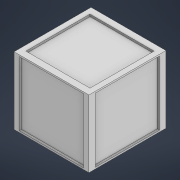
# Autodesk Inventor part: End-Effector
Saved by Autodesk Inventor 2022 (Build 260153000, 153)
## iProperties
Created: 2023-04-20
Part Number: End-Effector
Material: Generic
Document SubType Name: Modeling
Designer: Karl
Density: 1 g/cm^3
Appearance: Default
Author: Karl
Autodesk Inventor part; units mm, degrees
ref_plane "YZ Plane" through (0, 0, 0) normal (1, 0, 0) x (0, 1, 0)
ref_plane "XZ Plane" through (0, 0, 0) normal (0, 1, 0) x (-1, 0, 0)
ref_plane "XY Plane" through (0, 0, 0) normal (0, 0, 1) x (1, 0, 0)
sketch "Sketch3" plane through (0, 0, 0) normal (0, 0, 1) x (1, 0, 0)
  line L0 (0, 0) -> (-50, 0)
  line L1 (-50, 0) -> (-50, 43)
  line L2 (-50, 43) -> (0, 43)
  line L3 (0, 43) -> (0, 0)
  line L4 (10, -10) -> (-60, -10)
  line L5 (-60, -10) -> (-60, 53)
  line L6 (-60, 53) -> (10, 53)
  line L7 (10, 53) -> (10, -10)
  dimension "d26" = 43
  dimension "d27" = 50
  dimension "d28" = 70
  dimension "d29" = 63
  constraints: 16 end point, 4 parallel, 2 horizontal, 2 perpendicular
  measures "d26" distance of L2.end L0.start
  measures "d27" distance of L0.start L0.end
  measures "d28" distance of L5.end L6.end
  measures "d29" distance of L4.end L5.end
extrude "Extrusion3" add sketch "Sketch3" along normal blind 60
sketch "Sketch4" plane through (0, 0, 60) normal (0, 0, 1) x (1, 0, 0)
  line L0 (10, -10) -> (-60, -10)
  line L1 (-60, -10) -> (-60, 53)
  line L2 (-60, 53) -> (10, 53)
  line L3 (10, 53) -> (10, -10)
  point P0 (0, 0)
  constraints: 8 end point, 2 parallel, 1 horizontal, 1 perpendicular
extrude "Extrusion4" add sketch "Sketch4" along normal blind 12
sketch "Sketch5" plane through (-60, 53, 0) normal (0, 1, 0) x (1, 0, 0)
  line L0 (0, 0) -> (70, 0) projected
  line L1 (70, 0) -> (70, -72) projected
  line L2 (0, 0) -> (70, 0)
  line L3 (70, 0) -> (70, -72)
  line L4 (70, -72) -> (0, -72)
  line L5 (0, -72) -> (0, 0)
  line L6 (65, -6) -> (5, -6)
  line L7 (5, -6) -> (5, -66)
  line L8 (5, -66) -> (65, -66)
  line L9 (65, -66) -> (65, -6)
  line L10 (60, -11) -> (10, -11)
  line L11 (10, -11) -> (10, -61)
  line L12 (10, -61) -> (60, -61)
  line L13 (60, -61) -> (60, -11)
  point P0 (60, 0)
  dimension "d34" = 60
  dimension "d35" = 60
  dimension "d36" = 50
  dimension "d37" = 50
  constraints: 24 end point, 6 parallel, 3 horizontal, 3 perpendicular
  measures "d34" distance of L8.end L7.end
  measures "d35" distance of L7.end L6.end
  measures "d36" distance of L12.end L11.end
  measures "d37" distance of L11.end L10.end
extrude "Extrusion5" cut sketch "Sketch5" against normal blind 2 contours L9 L8 L7 L6 | L13 L12 L11 L10
sketch "Sketch6" plane through (10, -10, 0) normal (1, 0, 0) x (0, 0, -1)
  line L0 (-6, 1.5) -> (-66, 1.5)
  line L1 (-66, 1.5) -> (-66, 61.5)
  line L2 (-66, 61.5) -> (-6, 61.5)
  line L3 (-6, 61.5) -> (-6, 1.5)
  line L4 (-11, 6.5) -> (-61, 6.5)
  line L5 (-61, 6.5) -> (-61, 56.5)
  line L6 (-61, 56.5) -> (-11, 56.5)
  line L7 (-11, 56.5) -> (-11, 6.5)
  point P0 (0, 10)
  dimension "d40" = 60
  dimension "d41" = 60
  dimension "d42" = 50
  dimension "d43" = 50
  constraints: 16 end point, 4 parallel, 2 horizontal, 2 perpendicular
  measures "d40" distance of L1.end L2.end
  measures "d41" distance of L0.end L1.end
  measures "d42" distance of L5.end L6.end
  measures "d43" distance of L4.end L5.end
extrude "Extrusion6" cut sketch "Sketch6" against normal blind 2 contours L0 L1 L2 L3 | L4 L5 L6 L7
sketch "Sketch7" plane through (-60, -10, 0) normal (0, -1, 0) x (1, 0, 0)
  line L0 (5, 6) -> (65, 6)
  line L1 (65, 6) -> (65, 66)
  line L2 (65, 66) -> (5, 66)
  line L3 (5, 66) -> (5, 6)
  line L4 (10, 11) -> (60, 11)
  line L5 (60, 11) -> (60, 61)
  line L6 (60, 61) -> (10, 61)
  line L7 (10, 61) -> (10, 11)
  point P0 (60, 0)
  dimension "d46" = 60
  dimension "d47" = 60
  dimension "d48" = 50
  dimension "d49" = 50
  constraints: 16 end point, 4 parallel, 2 horizontal, 2 perpendicular
  measures "d46" distance of L2.end L1.end
  measures "d47" distance of L1.end L0.end
  measures "d48" distance of L6.end L5.end
  measures "d49" distance of L5.end L4.end
extrude "Extrusion7" cut sketch "Sketch7" against normal blind 2 contours L3 L2 L1 L0 | L7 L6 L5 L4
sketch "Sketch8" plane through (-60, -10, 0) normal (-1, 0, 0) x (0, 0, 1)
  line L0 (6, 1.5) -> (66, 1.5)
  line L1 (66, 1.5) -> (66, 61.5)
  line L2 (66, 61.5) -> (6, 61.5)
  line L3 (6, 61.5) -> (6, 1.5)
  line L4 (11, 6.5) -> (61, 6.5)
  line L5 (61, 6.5) -> (61, 56.5)
  line L6 (61, 56.5) -> (11, 56.5)
  line L7 (11, 56.5) -> (11, 6.5)
  point P0 (0, 10)
  dimension "d52" = 60
  dimension "d53" = 60
  dimension "d54" = 50
  dimension "d55" = 50
  constraints: 16 end point, 4 parallel, 2 horizontal, 2 perpendicular
  measures "d52" distance of L2.end L1.end
  measures "d53" distance of L1.end L0.end
  measures "d54" distance of L6.end L5.end
  measures "d55" distance of L5.end L4.end
extrude "Extrusion8" cut sketch "Sketch8" against normal blind 2 contours L3 L2 L1 L0 | L7 L6 L5 L4
sketch "Sketch9" plane through (0, 0, 72) normal (0, 0, 1) x (1, 0, 0)
  line L0 (5, -8.5) -> (-55, -8.5)
  line L1 (-55, -8.5) -> (-55, 51.5)
  line L2 (-55, 51.5) -> (5, 51.5)
  line L3 (5, 51.5) -> (5, -8.5)
  line L4 (0, 46.5) -> (-50, 46.5)
  line L5 (-50, 46.5) -> (-50, -3.5)
  line L6 (-50, -3.5) -> (0, -3.5)
  line L7 (0, -3.5) -> (0, 46.5)
  point P0 (0, 0)
  dimension "d58" = 60
  dimension "d59" = 60
  dimension "d60" = 50
  dimension "d61" = 50
  constraints: 16 end point, 4 parallel, 2 horizontal, 2 perpendicular
  measures "d58" distance of L1.end L2.end
  measures "d59" distance of L0.end L1.end
  measures "d60" distance of L6.end L5.end
  measures "d61" distance of L5.end L4.end
extrude "Extrusion9" cut sketch "Sketch9" against normal blind 2 contours L0 L1 L2 L3 | L7 L6 L5 L4
body "Solid2"
